Autodesk Fusion 360 part; units mm, degrees
(part 2 of 2)
sketch "Sketch12" plane through (0, 0, 37.5) normal (0, 0, 1) x (1, 0, 0)
  circle A0 centre (50, 0) radius 40
  dimension "d42" = 80
  measures "d42" diameter of A0
extrude "Extrude10" add sketch "Sketch12" along normal mid plane 21
sketch "Sketch13" plane through (0, 0, 27) normal (0, 0, -1) x (-1, 0, 0)
  line L0 (-10, 0.0146) -> (-90, 0.0146)
  arc A0 (-90, 0.0146) -> (-10, 0.0146) centre (-50, 0) ccw
  line L1 (-50, 0) -> (-50, -30)
  line L2 (-70, 0) -> (-70, -28.7228)
  line L3 (-30, 0) -> (-30, -28.7228)
  arc A1 (-70, -28.7228) -> (-30, -28.7228) centre (-50, 0) ccw
  dimension "d45" = 30
  dimension "d46" = 20
  dimension "d47" = -20
  dimension "d48" = 35
  constraint coincident A0.centre L1.start
  constraint perpendicular L0 L1
  measures "d45" distance of A0.centre L1.end
  measures "d48" radius of A1
sketch "Sketch14" plane through (0, 0, 27) normal (0, 0, -1) x (1, 0, 0)
  line L0 (70, 0) -> (50, 0)
  line L1 (50, 0) -> (30, 0)
  line L2 (30, 0) -> (30, 28.7225)
  line L3 (70, 0) -> (70, 28.7225)
  arc A0 (70, 28.7225) -> (30, 28.7225) centre (50, -0.3844) ccw
  constraint horizontal L0
  constraint parallel L0 L1
  constraint perpendicular L1 L2
  constraint perpendicular L1 L3
extrude "Extrude11" add sketch "Sketch14" along normal blind 35
sketch "Sketch15" plane through (135, 0, 0) normal (1, 0, 0) x (0, 0, -1)
sketch "Sketch16" plane through (70, 0, 0) normal (1, 0, 0) x (0, 0, -1)
  line L0 (-27, 0) -> (-27, -28.7225)
  line L1 (-27, -28.7225) -> (8, -28.7225)
  line L2 (8, -28.7225) -> (8, 0)
  line L3 (8, 0) -> (-27, 0)
sketch "Sketch17" plane through (70, 0, 0) normal (1, 0, 0) x (0, 0, -1)
sketch "Sketch18" plane through (70, 0, 0) normal (1, 0, 0) x (0, 0, -1)
move_body "Move5" bodies 1 to x (1, 0, 0) y (0, 1, 0) z (0, 0, 1) at (0, 0, 10)
sketch "Sketch19" plane through (70, 0, 0) normal (1, 0, 0) x (0, 0, -1)
move_body "Move6" bodies 1 to x (1, 0, 0) y (0, 1, 0) z (0, 0, 1) at (0, 0, -0.7)
sketch "Sketch20" plane through (70, 0, 0) normal (1, 0, 0) x (0, 0, -1)
move_body "Move7" bodies 1 to x (1, 0, 0) y (0, 1, 0) z (0, 0, 1) at (0, 0, -4)
move_body "Move8" bodies 1 to x (1, 0, 0) y (0, 1, 0) z (0, 0, 1) at (0, 0, -2)
sketch "Sketch21" plane through (70, 0, 0) normal (1, 0, 0) x (0, 0, -1)
move_body "Move9" bodies 1 to x (1, 0, 0) y (0, 1, 0) z (0, 0, 1) at (0, 0, 5)
sketch "Sketch22" plane through (70, 0, 0) normal (1, 0, 0) x (0, 0, -1)
  line L0 (-35.3, 0) -> (-35.3, -28.7225)
  line L1 (-35.3, -28.7225) -> (-0.3, -28.7225)
  line L2 (-0.3, -28.7225) -> (-0.3, 0)
  line L3 (-0.3, 0) -> (-35.3, 0)
  line L4 (0, 0) -> (0, -40)
  dimension "d54" = 40
  constraint coincident L4.start origin
  measures "d54" distance of L4.start L4.end
move_body "Move10" bodies 1 to x (1, 0, 0) y (0, 1, 0) z (0, 0, 1) at (0, 0, -0.3)
sketch "Sketch23" plane through (70, 0, 0) normal (1, 0, 0) x (0, 0, -1)
  line L0 (0, 0) -> (25, 0)
  arc A0 (0, -40) -> (25, 0) centre (-29.6341, 6.3338) ccw
  dimension "d55" = 25
  dimension "d56" = 55
  constraint coincident L0.start origin
  constraint horizontal L0
  measures "d55" distance of L0.start L0.end
  measures "d56" radius of A0
sketch "Sketch24" plane through (70, 0, 0) normal (1, 0, 0) x (0, 0, -1)
  line L0 (0, 0) -> (25, 0)
  line L1 (0, 0) -> (0, -40)
  arc A0 (0, -40) -> (25, 0) centre (-29.3089, 6.1306) ccw
  constraint coincident L0.start L1.start
  constraint horizontal L0
  constraint perpendicular L0 L1
extrude "Extrude12" add sketch "Sketch24" against normal blind 40
extrude "Extrude13" cut 1 faces at (50.7869, -38.2842, 0) along direction (0, 0, -1) blind 57
sketch "Sketch25" plane through (296, 0, 0) normal (1, 0, 0) x (0, 0, -1)
  circle A0 centre (-8, 43.0649) radius 32.384
  circle A1 centre (-8, 45.9847) radius 15
  dimension "d61" = 30
  measures "d61" diameter of A1
extrude "Extrude14" cut sketch "Sketch25" against normal blind 20 contours A1
sketch "Sketch26" plane through (0, 0, 56) normal (0, 0, 1) x (1, 0, 0)
  circle A0 centre (50, 0) radius 40
  circle A1 centre (50, 0) radius 15
  dimension "d64" = 30
  constraint concentric A0 A1
  measures "d64" diameter of A1
extrude "Extrude15" cut sketch "Sketch26" against normal blind 20 contours A1
equation "d43 = ( 21 / 2 ) * 1 mm"
